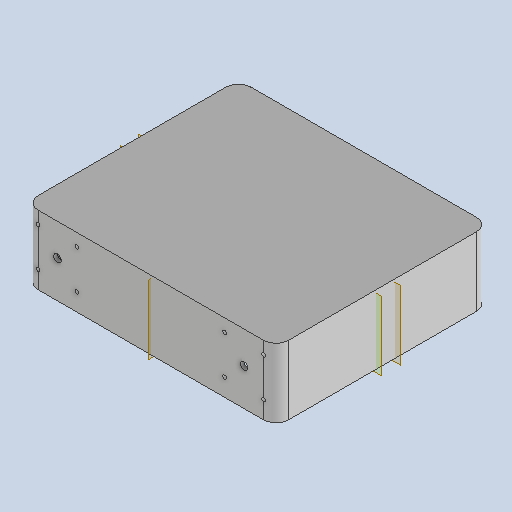
# Autodesk Inventor part: vozicek1
Saved by Autodesk Inventor 2024 (Build 280153000, 153)
## iProperties
Created: 2023-09-14
Part Number: vozicek1
Material: Generic
Document SubType Name: Modeling
Designer: jebes windows
Density: 1 g/cm^3
Appearance: Default
Author: jebes windows
## iProperties of the stored document vozicek1_3DPrint.ipt
Created: 2023-09-15
Part Number: vozicek1_3DPrint
Material: Generic
Document SubType Name: Modeling
Designer: jebes windows
Density: 1 g/cm^3
Appearance: Default
Author: jebes windows
Autodesk Inventor part; units mm, degrees
ref_plane "YZ Plane" through (0, 0, 0) normal (1, 0, 0) x (0, 1, 0)
ref_plane "XZ Plane" through (0, 0, 0) normal (0, 1, 0) x (-1, 0, 0)
ref_plane "XY Plane" through (0, 0, 0) normal (0, 0, 1) x (1, 0, 0)
ref_plane "Work Plane1" through (0, 0, 4.0499) normal (0, 0, 1) x (1, 0, 0)
sketch "Sketch1" plane through (0, 0, 4.0499) normal (0, 0, 1) x (1, 0, 0)
  arc A0 (7.5105, 16.375) -> (6.8105, 15.675) centre (7.5105, 15.675) ccw projected
  line L0 (0.7605, 16.375) -> (7.5105, 16.375) projected
  arc A1 (0.7605, 16.375) -> (-0.2395, 15.375) centre (0.7605, 15.375) ccw projected
  line L1 (-0.2395, 12.55) -> (-0.2395, 15.375) projected
  line L2 (0, 12.55) -> (-0.2395, 12.55) projected
  arc A2 (0, 12.55) -> (0.3941, 12.7423) centre (0, 13.05) ccw projected
  arc A3 (0.3941, 10.1577) -> (0.3941, 12.7423) centre (2.0494, 11.45) ccw projected
  arc A4 (0.3941, 10.1577) -> (0, 10.35) centre (0, 9.85) ccw projected
  line L3 (-0.2395, 10.35) -> (0, 10.35) projected
  line L4 (-0.2395, 2.7) -> (-0.2395, 10.35) projected
  line L5 (0, 2.7) -> (-0.2395, 2.7) projected
  arc A5 (0, 2.7) -> (0.3941, 2.8923) centre (0, 3.2) ccw projected
  arc A6 (0.3941, 0.3077) -> (0.3941, 2.8923) centre (2.0494, 1.6) ccw projected
  arc A7 (0.3941, 0.3077) -> (0, 0.5) centre (0, 0) ccw projected
  line L6 (-0.2395, 0.5) -> (0, 0.5) projected
  line L7 (-0.2395, -2.325) -> (-0.2395, 0.5) projected
  arc A8 (-0.2395, -2.325) -> (0.7605, -3.325) centre (0.7605, -2.325) ccw projected
  line L8 (7.5105, -3.325) -> (0.7605, -3.325) projected
  arc A9 (6.8105, -2.625) -> (7.5105, -3.325) centre (7.5105, -2.625) ccw projected
  line L9 (6.8105, 15.675) -> (6.8105, -2.625) projected
  line L10 (46.0105, -3.325) -> (7.5105, -3.325) projected
  line L11 (7.5105, 16.375) -> (46.0105, 16.375) projected
  arc A10 (46.0105, -3.325) -> (46.7105, -2.625) centre (46.0105, -2.625) ccw projected
  line L12 (52.7605, -3.325) -> (46.0105, -3.325) projected
  arc A11 (52.7605, -3.325) -> (53.7605, -2.325) centre (52.7605, -2.325) ccw projected
  line L13 (53.7605, 0.5) -> (53.7605, -2.325) projected
  line L14 (53.5211, 0.5) -> (53.7605, 0.5) projected
  arc A12 (53.5211, 0.5) -> (53.127, 0.3077) centre (53.5211, 0) ccw projected
  arc A13 (53.127, 2.8923) -> (53.127, 0.3077) centre (51.4717, 1.6) ccw projected
  arc A14 (53.127, 2.8923) -> (53.5211, 2.7) centre (53.5211, 3.2) ccw projected
  line L15 (53.7605, 2.7) -> (53.5211, 2.7) projected
  line L16 (53.7605, 10.35) -> (53.7605, 2.7) projected
  line L17 (53.5211, 10.35) -> (53.7605, 10.35) projected
  arc A15 (53.5211, 10.35) -> (53.127, 10.1577) centre (53.5211, 9.85) ccw projected
  arc A16 (53.127, 12.7423) -> (53.127, 10.1577) centre (51.4717, 11.45) ccw projected
  arc A17 (53.127, 12.7423) -> (53.5211, 12.55) centre (53.5211, 13.05) ccw projected
  line L18 (53.7605, 12.55) -> (53.5211, 12.55) projected
  line L19 (53.7605, 15.375) -> (53.7605, 12.55) projected
  arc A18 (53.7605, 15.375) -> (52.7605, 16.375) centre (52.7605, 15.375) ccw projected
  line L20 (46.0105, 16.375) -> (52.7605, 16.375) projected
  arc A19 (46.7105, 15.675) -> (46.0105, 16.375) centre (46.0105, 15.675) ccw projected
  line L21 (46.7105, -2.625) -> (46.7105, 15.675) projected
  circle A20 centre (51.4717, 11.45) radius 1.25
  circle A21 centre (51.4717, 1.6) radius 1.25
  line L22 (53.7605, 12.55) -> (53.7605, 10.35)
  line L23 (53.7605, 2.7) -> (53.7605, 0.5)
  line L24 (-0.2395, 12.55) -> (-0.2395, 10.35)
  line L25 (-0.2395, 2.7) -> (-0.2395, 0.5)
  circle A22 centre (2.0494, 1.6) radius 1.25
  circle A23 centre (2.0494, 11.45) radius 1.25
  line L26 (47.3105, 16.625) -> (6.3105, 16.625)
  line L27 (6.3105, 16.625) -> (6.3105, -3.875)
  line L28 (6.3105, -3.875) -> (47.3105, -3.875)
  line L29 (47.3105, -3.875) -> (47.3105, 16.625)
  line L30 (47.3105, 16.625) -> (6.3105, -3.875) construction
  line L31 (6.3105, 16.625) -> (47.3105, -3.875) construction
  point P0 (0, 0)
  point P1 (26.8105, 6.375)
  point P2 (6.8105, 6.525)
  point P3 (6.3105, -3.325)
  point P4 (6.3105, 16.375)
  point P5 (47.3105, 16.375)
  point P6 (47.3105, -3.325)
  dimension "d0" = 2.5
  dimension "d1" = 2.5
  dimension "d2" = 2.5
  dimension "d3" = 2.5
  dimension "d4" = 41
  dimension "d5" = 20.5
  dimension "d6" = 10
  dimension "d7" = 20
  constraints: 20 end point, 4 centre point, 4 coincident, 3 midpoint, 3 vertical, 2 parallel, 1 collinear, 1 horizontal, 1 perpendicular
  measures "d0" diameter of A20
  measures "d1" diameter of A21
  measures "d2" diameter of A22
  measures "d3" diameter of A23
  measures "d4" distance of L28.end L27.end
  measures "d5" distance of L27.end L26.end
  measures "d6" distance from line of L11 point (26.811, 6.375)
  measures "d7" horizontal distance of point (6.811, 6.525) point (26.811, 6.375)
extrude "Extrusion1" add sketch "Sketch1" along normal blind 40 contours L27 L8 A8 L7 L6 A7 A6 A5 L5 L4 L3 A4 A3 A2 L2 L1 A1 L0 | L20 A18 L19 L18 A17 A16 A15 L17 L16 L15 A14 A13 A12 L14 L13 A11 L12 L29 | L2 A2 A3 A4 L3 L24 | L25 L5 A5 A6 A7 L6 | L22 L17 A15 A16 A17 L18 | L14 A12 A13 A14 L15 L23
sketch "Sketch2" plane through (0, 0, 44.0499) normal (0, 0, 1) x (1, 0, 0)
  line L0 (-110.2395, 91.525) -> (89.7605, 91.525)
  line L1 (89.7605, 91.525) -> (89.7605, -78.475)
  line L2 (89.7605, -78.475) -> (-110.2395, -78.475)
  line L3 (-110.2395, -78.475) -> (-110.2395, 91.525)
  line L4 (-0.2395, 15.375) -> (-0.2395, -2.325) projected
  line L5 (-110.2395, 91.525) -> (89.7605, -78.475) construction
  line L6 (89.7605, 91.525) -> (-110.2395, -78.475) construction
  line L7 (-0.2395, 15.375) -> (-0.2395, -2.325) projected
  point P0 (0, 0)
  point P1 (-10.2395, 6.525)
  point P2 (-0.2395, 6.525)
  point P3 (-0.2395, 6.525)
  dimension "d10" = 200
  dimension "d11" = 170
  dimension "d111" = 10
  dimension "d112" = 0
  constraints: 12 end point, 3 midpoint, 2 parallel, 1 horizontal, 1 perpendicular
  measures "d10" distance of L1.end L2.end
  measures "d11" distance between parallel lines of L2 L0
  measures "d111" distance of point (-0.239, 6.525) point (-10.239, 6.525)
  measures "d112" vertical distance of point (-0.239, 6.525) point (-10.239, 6.525)
extrude "Extrusion2" add sketch "Sketch2" along normal blind 5
sketch "Sketch3" plane through (0, 0, 44.0499) normal (0, 0, -1) x (-1, 0, 0)
  arc A0 (0.2395, 15.375) -> (-0.7605, 16.375) centre (-0.7605, 15.375) ccw projected
  line L0 (0.2395, 15.375) -> (0.2395, -2.325) projected
  arc A1 (-0.7605, -3.325) -> (0.2395, -2.325) centre (-0.7605, -2.325) ccw projected
  line L1 (-0.7605, -3.325) -> (-6.3105, -3.325) projected
  line L2 (-6.3105, -3.325) -> (-6.3105, 16.375) projected
  line L3 (-6.3105, 16.375) -> (-0.7605, 16.375) projected
  arc A2 (-53.7605, -2.325) -> (-52.7605, -3.325) centre (-52.7605, -2.325) ccw projected
  line L4 (-53.7605, -2.325) -> (-53.7605, 15.375) projected
  arc A3 (-52.7605, 16.375) -> (-53.7605, 15.375) centre (-52.7605, 15.375) ccw projected
  line L5 (-52.7605, 16.375) -> (-47.3105, 16.375) projected
  line L6 (-47.3105, 16.375) -> (-47.3105, -3.325) projected
  line L7 (-47.3105, -3.325) -> (-52.7605, -3.325) projected
  line L8 (110.2395, -78.475) -> (-89.7605, -78.475) projected
  line L9 (110.2395, 91.525) -> (110.2395, -78.475) projected
  line L10 (-89.7605, 91.525) -> (110.2395, 91.525) projected
  line L11 (-89.7605, -78.475) -> (-89.7605, 91.525) projected
  line L12 (-84.7605, -73.475) -> (105.2395, -73.475)
  line L13 (105.2395, -73.475) -> (105.2395, 86.525)
  line L14 (105.2395, 86.525) -> (-84.7605, 86.525)
  line L15 (-84.7605, 86.525) -> (-84.7605, -73.475)
  point P0 (0, 0)
  dimension "d14" = 5
  constraints: 8 end point, 3 other
  measures "d14" distance between parallel lines of L8 L12
extrude "Extrusion3" add sketch "Sketch3" along normal blind 50 contours L8 L11 L10 L9
chamfer "Chamfer1" distance 5 angle 45 6 edges at (3.5355, 16.375, 44.0499) (0.0534, 16.0821, 44.0499) (-0.2395, 6.525, 44.0499) (0.0534, -3.0321, 44.0499) (3.5355, -3.325, 44.0499) (6.3105, 6.525, 44.0499)
chamfer "Chamfer2" distance 5 angle 45 6 edges at (53.7605, 6.525, 44.0499) (53.4676, 16.0821, 44.0499) (50.0355, 16.375, 44.0499) (53.4676, -3.0321, 44.0499) (50.0355, -3.325, 44.0499) (47.3105, 6.525, 44.0499)
fillet "Fillet5" radius 10 4 edges at (-110.2395, -78.475, 21.5499) (-110.2395, 91.525, 21.5499) (89.7605, -78.475, 21.5499) (89.7605, 91.525, 21.5499)
sketch "Sketch11" plane through (-105.2395, -73.475, 44.0499) normal (0, 1, 0) x (1, 0, 0)
  line L0 (5, 36) -> (36, 36)
  line L1 (36, 36) -> (36, 5)
  line L2 (36, 5) -> (5, 5)
  line L3 (5, 5) -> (5, 36)
  line L4 (5, 36) -> (36, 5) construction
  line L5 (36, 36) -> (5, 5) construction
  circle A0 centre (36, 36) radius 1.5
  circle A1 centre (5, 36) radius 1.5
  circle A2 centre (5, 5) radius 1.5
  circle A3 centre (36, 5) radius 1.5
  line L6 (5, -5) -> (185, -5) projected
  line L7 (-5, 50) -> (5, 50) projected
  line L8 (5, 50) -> (5, -5) projected
  line L9 (5, -5) -> (-5, -5) projected
  line L10 (-5, -5) -> (-5, 50) projected
  line L11 (0, 0) -> (0, 50) projected
  circle A4 centre (20.5, 20.5) radius 3
  point P0 (105.2395, 44.0499)
  dimension "d78" = 31
  dimension "d79" = 31
  dimension "d80" = 3
  dimension "d81" = 3
  dimension "d82" = 3
  dimension "d83" = 3
  dimension "d84" = 10
  dimension "d85" = 5
  dimension "d88" = 6
  constraints: 12 end point, 5 centre point, 5 coincident, 2 midpoint, 2 parallel, 1 horizontal, 1 perpendicular
  measures "d78" distance of L1.end L2.end
  measures "d79" distance of L0.end L1.end
  measures "d80" diameter of A0
  measures "d81" diameter of A1
  measures "d82" diameter of A2
  measures "d83" diameter of A3
  measures "d84" distance from line of L6 L1.end
  measures "d85" distance between parallel lines of L11 L3
  measures "d88" diameter of A4
extrude "Extrusion9" cut sketch "Sketch11" against normal blind 10 contours L8 A1 L0 | L0 A1 L3 | L3 A1 L8 | A0 L1 L0 | L0 L1 A0 | A2 L2 L3 | L3 L8 A2 | L2 A2 L8 | A3 L2 L1 | L1 L2 A3 | A4
ref_plane "Work Plane2" through (-105.2395, 16.525, 44.0499) normal (0, -1, 0) x (1, 0, 0)
ref_plane "Work Plane3" through (-10.2395, -73.475, 44.0499) normal (1, 0, 0) x (0, 0, -1)
mirror "Mirror2" about plane through (-10.2395, -73.475, 44.0499) normal (1, 0, 0) of "Extrusion9"
sketch "Sketch12" plane through (-105.2395, -73.475, 44.0499) normal (0, 1, 0) x (1, 0, 0)
  circle A0 centre (20.5, 20.5) radius 3 projected
  circle A1 centre (20.5, 20.5) radius 11
  point P0 (105.2395, 44.0499)
  dimension "d91" = 22
  constraints: 1 centre point, 1 coincident
  measures "d91" diameter of A1
extrude "Extrusion10" cut sketch "Sketch12" against normal blind 2
mirror "Mirror4" about plane through (-10.2395, -73.475, 44.0499) normal (1, 0, 0) of "Extrusion10"
ref_plane "Work Plane4" through (-105.2395, 1.525, 44.0499) normal (0, 1, 0) x (1, 0, 0)
mirror "Mirror5" about plane through (-105.2395, 1.525, 44.0499) normal (0, 1, 0) of "Extrusion9", "Extrusion10", "Mirror4", "Mirror2"
sketch "Sketch14" plane through (0, 0, 44.0499) normal (0, 0, -1) x (-1, 0, 0)
  line L0 (91.2395, -23.475) -> (16.2395, -23.475)
  line L1 (91.2395, 24.525) -> (8.2395, 24.525)
  circle A0 centre (16.2395, -23.475) radius 2.5
  circle A1 centre (16.2395, -23.475) radius 1.25
  circle A2 centre (91.2395, -23.475) radius 2.5
  circle A3 centre (91.2395, -23.475) radius 1.25
  circle A4 centre (8.2395, 24.525) radius 2.5
  circle A5 centre (8.2395, 24.525) radius 1.25
  circle A6 centre (91.2395, 24.525) radius 2.5
  circle A7 centre (91.2395, 24.525) radius 1.25
  line L2 (105.2395, 86.525) -> (105.2395, -73.475) projected
  line L3 (105.2395, -73.475) -> (-84.7605, -73.475) projected
  point P0 (0, 0)
  dimension "d97" = 5
  dimension "d98" = 2.5
  dimension "d99" = 5
  dimension "d100" = 2.5
  dimension "d101" = 5
  dimension "d102" = 2.5
  dimension "d103" = 5
  dimension "d104" = 2.5
  dimension "d105" = 75
  dimension "d106" = 83
  dimension "d107" = 48
  dimension "d108" = 14
  dimension "d109" = 14
  dimension "d110" = 50
  constraints: 8 centre point, 8 coincident, 4 end point, 2 horizontal
  measures "d97" diameter of A0
  measures "d98" diameter of A1
  measures "d99" diameter of A2
  measures "d100" diameter of A3
  measures "d101" diameter of A4
  measures "d102" diameter of A5
  measures "d103" diameter of A6
  measures "d104" diameter of A7
  measures "d105" distance of L0.start L0.end
  measures "d106" distance of L1.start L1.end
  measures "d107" distance of A6.centre L0.start
  measures "d108" distance from line of L2 L1.start
  measures "d109" distance from line of L2 L0.start
  measures "d110" distance between parallel lines of L3 L0
extrude "Extrusion11" add sketch "Sketch14" along normal blind 5
sketch "Sketch15" plane through (-110.2395, -68.475, -5.9501) normal (-1, 0, 0) x (0, 0, 1)
  line L0 (30.5, 51) -> (45.5, 51)
  line L1 (45.5, 51) -> (45.5, 66)
  line L2 (45.5, 66) -> (30.5, 66)
  line L3 (30.5, 66) -> (30.5, 51)
  line L4 (30.5, 51) -> (45.5, 66) construction
  line L5 (45.5, 51) -> (30.5, 66) construction
  line L6 (55, 0) -> (0, 0) projected
  line L7 (55, 150) -> (55, 0) projected
  line L8 (30.5, 82) -> (45.5, 82)
  line L9 (45.5, 82) -> (45.5, 94)
  line L10 (45.5, 94) -> (30.5, 94)
  line L11 (30.5, 94) -> (30.5, 82)
  line L12 (30.5, 82) -> (45.5, 94) construction
  line L13 (45.5, 82) -> (30.5, 94) construction
  point P0 (5.9501, 68.475)
  point P1 (38, 58.5)
  point P2 (38, 88)
  dimension "d115" = 15
  dimension "d116" = 15
  dimension "d117" = 58.5
  dimension "d118" = 17
  dimension "d121" = 15
  dimension "d122" = 12
  dimension "d123" = 0
  dimension "d124" = 29.5
  constraints: 24 end point, 4 midpoint, 4 parallel, 2 horizontal, 2 perpendicular
  measures "d115" distance of L2.end L1.end
  measures "d116" distance of L1.end L0.end
  measures "d117" distance from line of L6 point (38, 58.5)
  measures "d118" distance from line of L7 point (38, 58.5)
  measures "d121" distance of L10.end L9.end
  measures "d122" distance of L9.end L8.end
  measures "d123" horizontal distance of point (38, 58.5) point (38, 88)
  measures "d124" distance of point (38, 58.5) point (38, 88)
extrude "Extrusion12" cut sketch "Sketch15" against normal up to surface (5 mm away)
body "Solid1"
